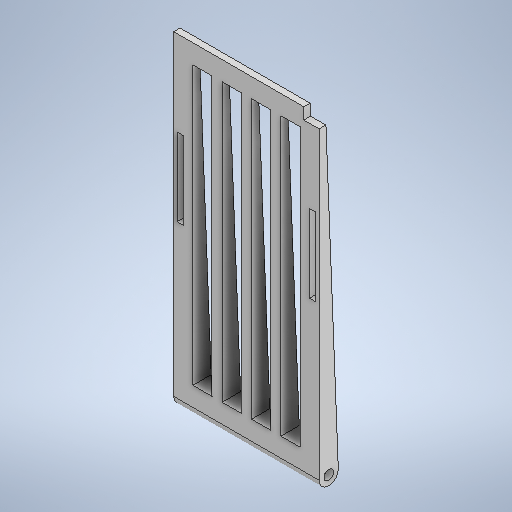
# Autodesk Inventor part: Ramp 2
Saved by Autodesk Inventor 2025.1 (Build 291241020, 241B)
## iProperties
Created: 2024-10-25
Part Number: Ramp 2
Material: Generic
Document SubType Name: Modeling
Designer: aly_g
Density: 1 g/cm^3
Appearance: Default
Author: aly_g
Autodesk Inventor part; units mm, degrees
ref_plane "YZ Plane" through (0, 0, 0) normal (1, 0, 0) x (0, 1, 0)
sketch "Sketch1" plane through (0, 0, 0) normal (0, 0, 1) x (1, 0, 0)
  line L0 (0, 170) -> (76, 170)
  line L1 (0, 0) -> (76, 0)
  line L2 (0, 170) -> (0, 0)
  line L3 (76, 170) -> (76, 0)
  point P0 (38, 170)
  point P1 (38, 0)
  dimension "d0" = 76
  dimension "d2" = 170
  constraints: 8 end point, 2 horizontal, 2 midpoint, 1 coincident, 1 parallel, 1 vertical alignment
  measures "d0" distance of L0.start L0.end
  measures "d2" distance of L1.start L0.start
extrude "Extrusion1" add sketch "Sketch1" along normal blind 10
fillet "Fillet1" radius 5 2 edges at (38, 0, 10) (38, 0, 0)
sketch "Sketch4" plane through (0, 5, 5) normal (-1, 0, 0) x (0, 0, 1)
  arc A0 (-5, 0) -> (5, 0) centre (0, 0) ccw projected
  line L0 (-5, 0) -> (2, 171.925)
  line L1 (-5, 0) -> (-5, 171.925)
  line L2 (-5, 171.925) -> (2, 171.925)
  line L3 (-5, 165) -> (-5, 0) projected
  point P0 (-5, -5)
  dimension "d22" = 171.925
  dimension "d23" = 7
  constraints: 6 end point, 2 perpendicular, 1 vertical
  measures "d22" distance of L1.end L0.start
  measures "d23" distance of L0.end L1.end
extrude "Extrusion3" cut sketch "Sketch4" against normal through all
sketch "Sketch5" plane through (0, 0, 10) normal (0, 0, 1) x (1, 0, 0)
  line L0 (10, 160) -> (20, 160)
  line L1 (20, 160) -> (20, 15)
  line L2 (20, 15) -> (10, 15)
  line L3 (10, 15) -> (10, 160)
  point P0 (0, 0)
  point P1 (15, 15)
  point P2 (15, 160)
  dimension "d26" = 15
  dimension "d27" = 10
  dimension "d28" = 160
  dimension "d29" = 10
  constraints: 8 end point, 2 midpoint, 2 parallel, 1 horizontal, 1 perpendicular
  measures "d26" horizontal distance of point (0, 0) point (15, 15)
  measures "d27" distance from line of point (0, 0) L3
  measures "d28" vertical distance of point (0, 0) point (15, 160)
  measures "d29" distance of L1.end L2.end
extrude "Extrusion4" cut sketch "Sketch5" against normal through all
pattern_linear "Rectangular Pattern1" count 4 spacing 15.3333 along (1, 0, 0) of "Extrusion4"
sketch "Sketch6" plane through (76, 5, 10) normal (1, 0, 0) x (0, 0, -1)
  arc A0 (0, 0) -> (10, 0) centre (5, 0) ccw projected
  line L0 (3, 1.5) -> (3, -1.5)
  arc A1 (3, -1.5) -> (3, 1.5) centre (5, 0) ccw
  point P0 (10, -5)
  point P1 (5, -5)
  dimension "d36" = 3
  dimension "d37" = 2.5
  constraints: 3 point on circle, 2 end point, 1 centre point, 1 concentric, 1 vertical
  measures "d36" distance of L0.end L0.start
  measures "d37" radius of A1
extrude "Extrusion5" cut sketch "Sketch6" against normal through all
sketch "Sketch8" plane through (0, 0, 10) normal (0, 0, 1) x (1, 0, 0)
  line L0 (74.25, 84.9) -> (70.95, 84.9)
  line L1 (70.95, 84.9) -> (70.95, 125.5)
  line L2 (70.95, 125.5) -> (74.25, 125.5)
  line L3 (74.25, 125.5) -> (74.25, 84.9)
  line L4 (76, 5) -> (0, 5) projected
  line L5 (58, 160) -> (58, 15) projected
  line L6 (76, 5) -> (76, 170) projected
  line L7 (76, 170) -> (0, 170) projected
  point P0 (0, 0)
  point P1 (72.6, 84.9)
  point P2 (72.6, 125.5)
  dimension "d43" = 3.3
  dimension "d45" = 79.9
  dimension "d49" = 1.75
  dimension "d59" = 40.6
  constraints: 8 end point, 2 midpoint, 2 parallel, 1 horizontal, 1 perpendicular
  measures "d43" distance of L1.end L2.end
  measures "d45" distance from line of L4 point (72.6, 84.9)
  measures "d49" distance from line of L6 L0.start
  measures "d59" distance of L0.end L1.end
extrude "Extrusion7" cut sketch "Sketch8" against normal through all
ref_plane "Work Plane1" through (38, 5, 10) normal (1, 0, 0) x (0, 0, -1)
ref_plane "Work Plane2" through (55.9999, 87.5, 0.4072) normal (0, 1, 0) x (1, 0, 0)
mirror "Mirror2" about plane through (38, 5, 10) normal (1, 0, 0) of "Extrusion7"
sketch "Sketch9" plane through (0, 0, 10) normal (0, 0, 1) x (1, 0, 0)
  line L0 (68, 170) -> (76, 170)
  line L1 (76, 170) -> (76, 164)
  line L2 (76, 164) -> (68, 164)
  line L3 (68, 164) -> (68, 170)
  point P0 (0, 0)
  point P1 (76, 167)
  point P2 (76, 5)
  point P3 (72, 170)
  point P4 (0, 170)
  dimension "d50" = 8
  dimension "d51" = 6
  constraints: 8 end point, 2 midpoint, 2 parallel, 1 horizontal, 1 horizontal alignment, 1 perpendicular, 1 vertical alignment
  measures "d50" distance of L1.end L2.end
  measures "d51" distance of point (76, 170) L1.end
extrude "Extrusion8" cut sketch "Sketch9" against normal through all
sketch "Sketch10" plane through (0, 5, 10) normal (-1, 0, 0) x (0, 0, 1)
  arc A0 (-3, 1.5) -> (-3, -1.5) centre (-5, 0) ccw projected
  circle A1 centre (-5, 0) radius 2.5
  arc A2 (-10, 0) -> (0, 0) centre (-5, 0) ccw projected
  point P0 (-10, -5)
  point P1 (-5, -5)
  point P2 (-3, -1.5)
  point P3 (-3, 1.5)
  dimension "d58" = 5
  constraints: 1 centre point, 1 coincident, 1 point on circle, 1 vertical alignment
  measures "d58" diameter of A1
extrude "Extrusion9" cut sketch "Sketch10" against normal blind 4
body "Solid1"
